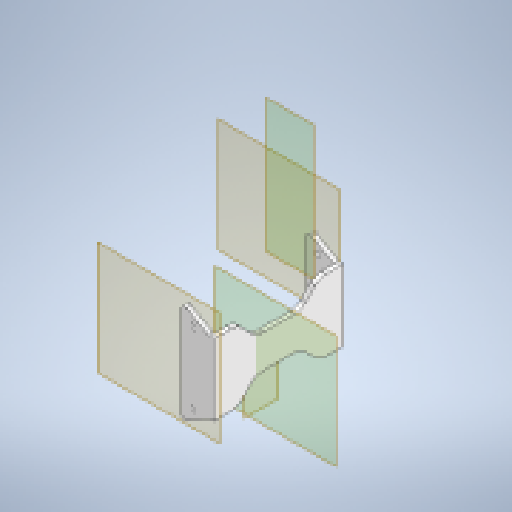
# Autodesk Inventor part: 부품30
Saved by Autodesk Inventor 2024.3 (Build 283343000, 343)
## iProperties
Created: 2024-09-06
Part Number: 부품30
Material: LCP 플라스틱
Document SubType Name: Modeling
Designer: 구지현
Density: 1.626 g/cm^3
Appearance: 매끄러움 - 흰색
Mass: 20.9856 g
Surface Area: 99.6171 cm^2
Volume: 12.9063 cm^3
Author: 구지현
Autodesk Inventor part; units mm, degrees
ref_plane "YZ Plane" through (0, 0, 0) normal (1, 0, 0) x (0, 1, 0)
ref_plane "XZ Plane" through (0, 0, 0) normal (0, 1, 0) x (-1, 0, 0)
ref_plane "XY Plane" through (0, 0, 0) normal (0, 0, 1) x (1, 0, 0)
ref_plane "작업 평면1" through (0, 0, -70) normal (0, 0, 1) x (-1, 0, 0)
ref_plane "작업 평면2" through (73.607175, -5.321073, 6) normal (0, 0, -1) x (-1, 0, 0)
ref_plane "작업 평면3" through (33.563527, 47.68984, -43) normal (0, 0, -1) x (-0.0000002, -1, 0)
sketch "스케치2" plane through (48.6072, 47.68984, -49) normal (0, 0, 1) x (0.0000002, -1, 0)
  arc A0 (22.242963, -4.320506) -> (23.975013, -7.320506) centre (23.975013, -5.320506) ccw
  line L0 (30.510915, 10) -> (22.242963, -4.320506)
  line L1 (75.510915, 9.999992) -> (30.510915, 10)
  line L2 (83.778861, -4.320518) -> (75.510915, 9.999992)
  arc A1 (82.04681, -7.320517) -> (83.778861, -4.320518) centre (82.04681, -5.320517) ccw
  line L3 (23.975013, -7.320506) -> (82.04681, -7.320517)
  circle A2 centre (30.510913, -0.000009) radius 1.65
  circle A3 centre (75.510913, -0.000008) radius 1.65
  point P0 (47.689831, -48.607209)
extrude "돌출2" add sketch "스케치2" along normal blind 3
ref_plane "작업 평면4" through (58.607206, -27.821073, 0) normal (1, 0, 0) x (0, 0, -1)
ref_plane "작업 평면5" through (23.607206, -5.321073, 30) normal (0, 0, 1) x (-1, 0, 0)
sketch "스케치4" plane through (23.607206, -5.321073, 30) normal (0, 0, 1) x (-1, 0, 0)
  line L0 (-17.679492, -29.035898) -> (-17.679492, 29.035898)
  arc A0 (-20.679492, -30.767949) -> (-17.679492, -29.035898) centre (-19.679492, -29.035898) ccw
  line L1 (-35, -22.5) -> (-20.679492, -30.767949)
  line L2 (-20.679492, 30.767949) -> (-35, 22.5)
  arc A1 (-17.679492, 29.035898) -> (-20.679492, 30.767949) centre (-19.679492, 29.035898) ccw
  circle A2 centre (-25, 22.5) radius 1.65
  circle A3 centre (-24.99999, -22.5) radius 1.65
  line L3 (-35, 22.5) -> (-35, -22.5)
  point P0 (23.607206, -5.321073)
extrude "돌출4" add sketch "스케치4" along normal blind 3
sketch "스케치5" plane through (58.607206, -27.821073, -49) normal (1, 0, 0) x (0, 0, -1)
  line L0 (0, 0) -> (0, 45) projected
  line L1 (0, 45) -> (-3, 45) projected
  line L2 (-3, 0) -> (-3, 45) projected
  line L3 (0, 0) -> (-3, 0) projected
  line L4 (-79, 0) -> (-79, 45) projected
  line L5 (-79, 45) -> (-82, 45) projected
  line L6 (-82, 0) -> (-82, 45) projected
  line L7 (-79, 0) -> (-82, 0) projected
  line L8 (0, 0) -> (-82, 0)
  line L9 (-82, 0) -> (-82, 45)
  line L10 (-82, 45) -> (0, 45)
  line L11 (0, 45) -> (0, 0)
  point P0 (-49, 27.821073)
  point P1 (-79, 0)
  constraints: 8 end point, 2 parallel, 1 horizontal, 1 perpendicular
extrude "돌출5" add sketch "스케치5" along normal blind 3
sketch "스케치6" plane through (61.607206, -27.821073, -49) normal (1, 0, 0) x (0, 0, -1)
  line L0 (0, 0) -> (0, 45)
  line L1 (0, 45) -> (-82, 45)
  line L2 (-82, 45) -> (-82, 0)
  line L3 (-82, 0) -> (0, 0)
  line L4 (-67, 43.221829) -> (-73, 43.221829)
  line L5 (-67, 43.221829) -> (-67, 113.722149)
  line L6 (-67, 113.722149) -> (-73, 113.722149)
  line L7 (-73, 43.221829) -> (-73, 113.722149)
  line L8 (-73, 1.778179) -> (-67, 1.778179)
  line L9 (-73, -68.722141) -> (-73, 1.778179)
  line L10 (-67, -68.722141) -> (-73, -68.722141)
  line L11 (-67, -68.722141) -> (-67, 1.778179)
  line L12 (-15, 1.778178) -> (-9, 1.778178)
  line L13 (-15, 1.778178) -> (-15, -68.722142)
  line L14 (-15, -68.722142) -> (-9, -68.722142)
  line L15 (-9, 1.778178) -> (-9, -68.722142)
  line L16 (-9, 43.221829) -> (-15, 43.221829)
  line L17 (-9, 113.722149) -> (-9, 43.221829)
  line L18 (-15, 113.722149) -> (-9, 113.722149)
  line L19 (-15, 113.722149) -> (-15, 43.221829)
  line L20 (-67, 45) -> (-15, 45)
  line L21 (-15, 45) -> (-15, 33)
  line L22 (-15, 33) -> (-67, 33)
  line L23 (-67, 33) -> (-67, 45)
  line L24 (-67, 0) -> (-15, 0)
  line L25 (-15, 0) -> (-15, 12)
  line L26 (-15, 12) -> (-67, 12)
  line L27 (-67, 12) -> (-67, 0)
  point P0 (-49, 27.821073)
  point P1 (-67, 1.778179)
  point P2 (-15, 0)
  point P3 (-15, 1.778178)
  point P4 (-15, 43.221829)
  point P5 (-15, 45)
  dimension "d21" = 12
  dimension "d22" = 12
  constraints: 16 end point, 5 point on line, 4 parallel, 2 horizontal, 2 perpendicular
  measures "d21" distance of L20.end L21.end
  measures "d22" distance of L25.end L24.end
extrude "돌출6" cut sketch "스케치6" against normal blind 10 contours L3 L11 L27 L26 L25 L13 | L19 L21 L22 L23 L5 L1
chamfer "모따기1" distance 12 angle 45 4 edges at (60.1072, 5.1789, -34) (60.1072, 5.1789, 18) (60.1072, -15.8211, 18) (60.1072, -15.8211, -34)
fillet "모깎기1" radius 10 20 edges at (61.6072, 17.1789, 18) (60.1072, 17.1789, 18) (60.1072, 17.1788, 18) (58.6072, 17.1789, 18) (60.1072, 5.1789, 6.0001) (60.1072, 5.1789, -22.0001) (61.6072, 17.1789, -34) (60.1072, 17.1789, -34) (58.6072, 17.1789, -34) (60.1072, 17.1788, -34) (60.1072, -15.8211, -22.0001) (60.1072, -15.8211, 6.0001) (61.6072, -27.821, 18) (60.1072, -27.821, 18) (58.6072, -27.821, 18) (60.1072, -27.8211, 18) (61.6072, -27.821, -34) (58.6072, -27.821, -34) (60.1072, -27.821, -34) (60.1072, -27.8211, -34)
